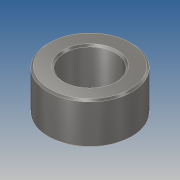
# Autodesk Inventor part: 200-60-DIFFERENTIAL-BAR-04
Saved by Autodesk Inventor 2018.2 (Build 222227000, 227)
## iProperties
Manager: feesmrt
Company: FRANCOR
Part Number: 200-60-DIFFERENTIAL-BAR-04
Project: Rescue Robot
Cost Center: -
Material: Edelstahl
Document SubType Name: Modeling
Designer: feesmrt
Engineer: feesmrt
Authority: feesmrt
Density: 8 g/cm^3
Appearance: Halbpoliert
Description: Differential Distanzhülse
Stock Number: 200-60-DIFFERENTIAL-BAR-04
Subject: Rescue Robot
Author: feesmrt
Revision Number: 1
Title: Differential Distanzhülse
Autodesk Inventor part; units mm, degrees
ref_plane "YZ Plane" through (0, 0, 0) normal (1, 0, 0) x (0, 1, 0)
ref_plane "XZ Plane" through (0, 0, 0) normal (0, 1, 0) x (-1, 0, 0)
ref_plane "XY Plane" through (0, 0, 0) normal (0, 0, 1) x (1, 0, 0)
sketch "Skizze2" plane through (0, 0, 0) normal (0, 0, 1) x (1, 0, 0)
  line L0 (-7, 0) -> (7, 0) projected
  line L1 (0, 7) -> (0, -7) projected
  circle A0 centre (0, 0) radius 5
  circle A1 centre (0, 0) radius 3.05
  dimension "d13" = 10
  dimension "d14" = 6.1
  constraints: 2 centre point, 2 coincident
  measures "d13" diameter of A0
  measures "d14" diameter of A1
extrude "Grundkörper" add sketch "Skizze2" along normal mid plane 5 contours A1 L1 A0 L0 | L0 A0 L1 A1 | A1 L0 A0 L1 | L1 A0 L0 A1
chamfer "Fase_Allgemein" distance 0.2 angle 45 4 edges at (-3.05, 0, 2.5) (-5, 0, 2.5) (-3.05, 0, -2.5) (-5, 0, -2.5)
